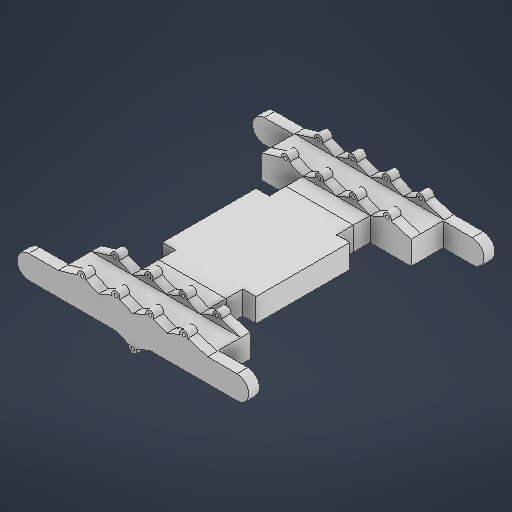
# Autodesk Inventor part: Base Plate
Saved by Autodesk Inventor 2026.3 (Build 303398000, 398)
## iProperties
Created: 2026-06-22
Part Number: Base Plate
Material: Generic
Document SubType Name: Modeling
Designer: Inigo Greenall
Density: 1 g/cm^3
Appearance: Default
Author: Inigo Greenall
Autodesk Inventor part; units mm, degrees
sketch "Sketch1" plane through (0, 0, 0) normal (0, 1, 0) x (-1, 0, 0)
  line L0 (98.75, 105) -> (-98.75, 105)
  line L1 (-98.75, 105) -> (-98.75, -105)
  line L2 (-98.75, -105) -> (98.75, -105)
  line L3 (98.75, -105) -> (98.75, 105)
  line L4 (98.75, 95.75) -> (63.75, 95.75)
  line L5 (63.75, 95.75) -> (63.75, -95.75)
  line L6 (63.75, -95.75) -> (98.75, -95.75)
  line L7 (-98.75, 95.75) -> (-63.75, 95.75)
  line L8 (-63.75, 95.75) -> (-63.75, -95.75)
  line L9 (-63.75, -95.75) -> (-98.75, -95.75)
  line L10 (63.75, 68.5) -> (-63.75, 68.5)
  line L11 (-63.75, 68.5) -> (-63.75, -68.5)
  line L12 (-63.75, -68.5) -> (63.75, -68.5)
  line L13 (63.75, -68.5) -> (63.75, 68.5)
  line L14 (28.75, 68.5) -> (28.75, -68.5)
  line L15 (-28.75, 68.5) -> (-28.75, -68.5)
  line L16 (0, -40) -> (40, -40)
  line L17 (40, -40) -> (40, 40)
  line L18 (40, 40) -> (-40, 40)
  line L19 (-40, 40) -> (-40, -40)
  line L20 (-40, -40) -> (0, -40)
  point P0 (0, 0)
  point P1 (98.75, 0)
  point P2 (0, 105)
  point P3 (-63.75, 0)
  point P4 (63.75, 0)
  point P5 (-63.75, 68.5)
  point P6 (63.75, -68.5)
  point P7 (0, 40)
  point P8 (40, 0)
  point P9 (-40, 0)
  point P10 (-28.75, -40)
  point P11 (-28.75, 40)
  point P12 (28.75, 40)
  point P13 (28.75, -40)
  dimension "d2" = 210
  dimension "d5" = 35
  dimension "d6" = 35
  dimension "d7" = 191.5
  dimension "d8" = 191.5
  dimension "d9" = 197.5
  dimension "d80" = 36.5
  dimension "d81" = 36.5
  dimension "d82" = 70
  dimension "d83" = 70
  dimension "d100" = 80
  dimension "d101" = 80
  constraints: 42 end point, 12 perpendicular, 11 point on line, 7 midpoint, 5 horizontal alignment, 4 horizontal, 4 parallel, 3 vertical alignment
  measures "d2" distance between parallel lines of L2 L0
  measures "d5" distance between parallel lines of L5 L3
  measures "d6" distance between parallel lines of L1 L8
  measures "d7" distance between parallel lines of L6 L4
  measures "d8" distance between parallel lines of L9 L7
  measures "d9" distance of L0.start L0.end
  measures "d80" distance between parallel lines of L0 L10
  measures "d81" distance between parallel lines of L2 L12
  measures "d82" distance between parallel lines of L14 L3
  measures "d83" distance between parallel lines of L15 L1
  measures "d100" distance of L16.end L17.end
  measures "d101" distance of L17.end L18.end
extrude "Extrusion1" add sketch "Sketch1" along normal blind 20 contours L3 L4 L5 L10 L8 L7 L1 L0 | L3 L2 L1 L9 L8 L12 L5 L6 | L14 L18 L15 L10 | L12 L15 L20 L16 L14 | L18 L17 L16 L14 | L14 L16 L20 L15 L18 | L15 L20 L19 L18
fillet "Fillet1" radius 10 8 edges at (98.75, 20, 100.375) (98.75, 0, 100.375) (-98.75, 20, 100.375) (-98.75, 0, 100.375) (-98.75, 0, -100.375) (-98.75, 20, -100.375) (98.75, 20, -100.375) (98.75, 0, -100.375)
ref_plane "Work Plane1" through (-88.75, 0, 88.875) normal (0, 0, 1) x (1, 0, 0)
sketch "Sketch6" plane through (-88.75, 0, 105) normal (0, 0, 1) x (1, 0, 0)
  line L0 (0, 0) -> (177.5, 0)
  arc A0 (177.5, 0) -> (177.5, 20) centre (177.5, 10) ccw projected
  line L1 (25, 0) -> (25, 20) projected
  arc A1 (0, 20) -> (0, 0) centre (0, 10) ccw projected
  line L2 (0, 20) -> (177.5, 20)
  line L3 (152.5, 0) -> (152.5, 20) projected
  circle A2 centre (45.25, 26.05) radius 1.5
  circle A3 centre (74.25, 26.05) radius 1.5
  circle A4 centre (103.25, 26.05) radius 1.5
  circle A5 centre (132.25, 26.05) radius 1.5
  line L4 (0, 20) -> (177.5, 20) projected
  line L5 (45.25, 26.05) -> (132.25, 26.05)
  line L6 (132.25, 26.05) -> (152.5, 20)
  line L7 (25, 0) -> (25, 20) projected
  line L8 (45.25, 26.05) -> (25, 20)
  circle A6 centre (45.25, 26.05) radius 3.5
  circle A7 centre (74.25, 26.05) radius 3.5
  circle A8 centre (103.25, 26.05) radius 3.5
  circle A9 centre (132.25, 26.05) radius 3.5
  line L9 (45.25, 26.05) -> (59.75, 20)
  line L10 (59.75, 20) -> (74.25, 26.05)
  line L11 (74.25, 26.05) -> (88.75, 20)
  line L12 (88.75, 20) -> (103.25, 26.05)
  line L13 (103.25, 26.05) -> (117.75, 20)
  line L14 (117.75, 20) -> (132.25, 26.05)
  point P0 (88.75, 0)
  point P1 (135.6035, 25.0481)
  point P2 (128.75, 26.05)
  point P3 (130.75, 26.05)
  point P4 (133.6872, 25.6206)
  point P5 (106.75, 26.05)
  point P6 (99.75, 26.05)
  point P7 (101.75, 26.05)
  point P8 (104.75, 26.05)
  point P9 (77.75, 26.05)
  point P10 (70.75, 26.05)
  point P11 (72.75, 26.05)
  point P12 (75.75, 26.05)
  point P13 (48.75, 26.05)
  point P14 (41.8965, 25.0481)
  point P15 (43.8128, 25.6206)
  point P16 (46.75, 26.05)
  point P17 (129.0199, 24.7023)
  point P18 (106.4801, 24.7023)
  point P19 (100.0199, 24.7023)
  point P20 (77.4801, 24.7023)
  point P21 (71.0199, 24.7023)
  point P22 (48.4801, 24.7023)
  dimension "d61" = 3
  dimension "d62" = 2
  dimension "d63" = 6.05
  dimension "d64" = 29
  dimension "d65" = 29
  dimension "d66" = 29
  dimension "d67" = 45.25
  constraints: 22 end point, 8 centre point, 6 equal radius, 4 coincident, 3 parallel, 3 point on line, 2 horizontal, 1 equal length, 1 midpoint
  measures "d61" diameter of A2
  measures "d62" radial gap between concentric circles of A6 A2
  measures "d63" distance between parallel lines of L2 L5
  measures "d64" distance of A3.centre L9.start
  measures "d65" distance of A4.centre L10.end
  measures "d66" distance of L5.end A4.centre
  measures "d67" horizontal distance of L5.start L2.start
extrude "Extrusion5" add sketch "Sketch6" against normal up to surface (36.5 mm away) contours L8 A6 L9 L2 | L2 L14 A9 L6 | L10 A7 L11 L2 | A6 L5 A2 L8 | L8 A2 L9 A6 | L2 L12 A8 L13 | A9 L14 A5 L6 | L6 A5 L5 A9 | L9 A2 L5 A6 | L10 A3 L11 A7 | A7 L5 A3 L10 | L13 A4 L5 A8 | A8 L12 A4 L13 | A9 L5 A5 L14 | L11 A3 L5 A7 | A8 L5 A4 L12 | A7 L5 A3 | L5 A4 A8
ref_plane "Work Plane5" through (-88.75, 0, 91.75) normal (0, 0, 1) x (1, 0, 0)
sketch "Sketch11" plane through (-88.75, 0, 105) normal (0, 0, 1) x (1, 0, 0)
  circle A0 centre (88.75, -6.05) radius 3.5
  circle A1 centre (88.75, -6.05) radius 1.5
  line L0 (88.75, -6.05) -> (74.2515, 0)
  line L1 (0, 0) -> (177.5, 0) projected
  line L2 (88.75, -6.05) -> (103.2485, 0)
  point P0 (88.75, 0)
  point P1 (88.75, 0)
  point P2 (91.9801, -4.7021)
  point P3 (85.5199, -4.7021)
  dimension "d91" = 7
  dimension "d93" = 134.7
  dimension "d94" = 6.05
  dimension "d97" = 2
  constraints: 4 end point, 2 centre point, 2 point on line, 1 coincident, 1 equal length, 1 midpoint, 1 vertical alignment
  measures "d91" diameter of A0
  measures "d93" angle of L2 L0
  measures "d94" distance from line of L1 A0.centre
  measures "d97" radial gap between concentric circles of A1 A0
extrude "Extrusion7" add sketch "Sketch11" against normal up to surface (36.5 mm away) contours A0 L0 A1 L2 | L2 A1 L0 A0 | A0 L0 L1 L2
sketch "Sketch10" plane through (-88.75, 0, 91.75) normal (0, 0, 1) x (1, 0, 0)
  arc A0 (48.4801, 24.7023) -> (41.8965, 25.0481) centre (45.25, 26.05) ccw projected
  arc A1 (77.4801, 24.7023) -> (71.0199, 24.7023) centre (74.25, 26.05) ccw projected
  arc A2 (106.4801, 24.7023) -> (100.0199, 24.7023) centre (103.25, 26.05) ccw projected
  arc A3 (135.6035, 25.0481) -> (129.0199, 24.7023) centre (132.25, 26.05) ccw projected
  circle A4 centre (45.25, 26.05) radius 1.5 projected
  circle A5 centre (74.25, 26.05) radius 1.5 projected
  circle A6 centre (103.25, 26.05) radius 1.5 projected
  circle A7 centre (132.25, 26.05) radius 1.5 projected
  circle A8 centre (74.25, 26.05) radius 3.5
  line L0 (117.75, 20) -> (106.4801, 24.7023) projected
  circle A9 centre (103.25, 26.05) radius 3.5
  circle A10 centre (132.25, 26.05) radius 3.5
  circle A11 centre (45.25, 26.05) radius 3.5
  circle A12 centre (88.75, -6.05) radius 1.5 projected
  arc A13 (85.5199, -4.7021) -> (91.9801, -4.7021) centre (88.75, -6.05) ccw projected
  circle A14 centre (88.75, -6.05) radius 3.5
  line L1 (91.9801, -4.7021) -> (103.2485, 0) projected
  line L2 (74.2515, 0) -> (85.5199, -4.7021) projected
  line L3 (103.2485, 0) -> (74.2515, 0) projected
  line L4 (129.0199, 24.7023) -> (117.75, 20) projected
  line L5 (117.75, 20) -> (106.4801, 24.7023) projected
  line L6 (100.0199, 24.7023) -> (88.75, 20) projected
  line L7 (88.75, 20) -> (77.4801, 24.7023) projected
  line L8 (71.0199, 24.7023) -> (59.75, 20) projected
  line L9 (59.75, 20) -> (48.4801, 24.7023) projected
  line L10 (41.8965, 25.0481) -> (25, 20) projected
  line L11 (25, 20) -> (60, 20) projected
  line L12 (60, 20) -> (88.75, 20) projected
  line L13 (88.75, 20) -> (117.5, 20) projected
  line L14 (117.5, 20) -> (60, 20) projected
  line L15 (152.5, 20) -> (135.6035, 25.0481) projected
  line L16 (88.75, 20) -> (117.5, 20)
  line L17 (117.5, 20) -> (152.5, 20)
  point P0 (129.0199, 24.7023)
  point P1 (91.9801, -4.7021)
  point P2 (100.0199, 24.7023)
  point P3 (41.8965, 25.0481)
  point P4 (91.9801, -4.7021)
  point P5 (129.0199, 24.7023)
  constraints: 5 coincident, 4 end point, 2 collinear, 15 other
extrude "Extrusion6" cut sketch "Sketch10" along normal blind 5 and the other way blind 15
mirror "Mirror1" about plane through (0, 0, 0) normal (0, 0, 1) of "Extrusion5", "Extrusion6", "Extrusion7"
ref_plane "Work Plane8" through (-28.75, 0, 54.25) normal (0, 0, -1) x (-1, 0, 0)
ref_plane "Work Plane9" through (-28.75, 0, -54.25) normal (0, 0, -1) x (-1, 0, 0)
split body "Split8" result two bodies by plane through (-28.75, 0, 54.25) normal (0, 0, -1) first body at (-9.5833, 0.5, -13.3333)
split body "Split9" result two bodies by plane through (-28.75, 0, -54.25) normal (0, 0, -1) bodies 2 first body at (-35.6662, 0.5, -87)
equation "\"d6\" = d5"
equation "\"d8\" = d7"
body "Solid9"
body "Solid10"
body "Solid11"
